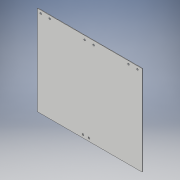
# Autodesk Inventor part: side shield
Saved by Autodesk Inventor 2017 (Build 210142000, 142)
## iProperties
Created: 2017-06-15
Part Number: side shield
Material: Generic
Document SubType Name: Modeling
Designer: slong
Density: 1 g/cm^3
Appearance: Default
Author: slong
Autodesk Inventor part; units mm, degrees
ref_plane "YZ Plane" through (0, 0, 0) normal (1, 0, 0) x (0, 1, 0)
ref_plane "XZ Plane" through (0, 0, 0) normal (0, 1, 0) x (-1, 0, 0)
ref_plane "XY Plane" through (0, 0, 0) normal (0, 0, 1) x (1, 0, 0)
sketch "Sketch1" plane through (0, 0, 0) normal (0, 0, 1) x (1, 0, 0)
  line L0 (0, -381) -> (0, 0)
  line L1 (0, 0) -> (444.5, 0)
  line L2 (444.5, 0) -> (444.5, -381)
  line L3 (444.5, -381) -> (0, -381)
  spline S0 degree 3 poles (17.3867, -12.7) (17.3867, -14.6709) (15.7889, -16.2687) (13.818, -16.2687) (11.847, -16.2687) (10.2493, -14.6709) (10.2493, -12.7) (10.2493, -10.7291) (11.847, -9.1313) (13.818, -9.1313) (15.7889, -9.1313) (17.3867, -10.7291) (17.3867, -12.7) knots 0 0 0 0 1 1 1 2 2 2 3 3 3 4 4 4 4
  line L4 (17.3867, -12.7) -> (17.3867, -14.6709) construction
  line L5 (17.3867, -14.6709) -> (15.7889, -16.2687) construction
  line L6 (15.7889, -16.2687) -> (13.818, -16.2687) construction
  line L7 (13.818, -16.2687) -> (11.847, -16.2687) construction
  line L8 (11.847, -16.2687) -> (10.2493, -14.6709) construction
  line L9 (10.2493, -14.6709) -> (10.2493, -12.7) construction
  line L10 (10.2493, -12.7) -> (10.2493, -10.7291) construction
  line L11 (10.2493, -10.7291) -> (11.847, -9.1313) construction
  line L12 (11.847, -9.1313) -> (13.818, -9.1313) construction
  line L13 (13.818, -9.1313) -> (15.7889, -9.1313) construction
  line L14 (15.7889, -9.1313) -> (17.3867, -10.7291) construction
  line L15 (17.3867, -10.7291) -> (17.3867, -12.7) construction
  spline S1 degree 3 poles (55.4867, -12.7) (55.4867, -14.6709) (53.8889, -16.2687) (51.918, -16.2687) (49.947, -16.2687) (48.3493, -14.6709) (48.3493, -12.7) (48.3493, -10.7291) (49.947, -9.1313) (51.918, -9.1313) (53.8889, -9.1313) (55.4867, -10.7291) (55.4867, -12.7) knots 0 0 0 0 1 1 1 2 2 2 3 3 3 4 4 4 4
  line L16 (55.4867, -12.7) -> (55.4867, -14.6709) construction
  line L17 (55.4867, -14.6709) -> (53.8889, -16.2687) construction
  line L18 (53.8889, -16.2687) -> (51.918, -16.2687) construction
  line L19 (51.918, -16.2687) -> (49.947, -16.2687) construction
  line L20 (49.947, -16.2687) -> (48.3493, -14.6709) construction
  line L21 (48.3493, -14.6709) -> (48.3493, -12.7) construction
  line L22 (48.3493, -12.7) -> (48.3493, -10.7291) construction
  line L23 (48.3493, -10.7291) -> (49.947, -9.1313) construction
  line L24 (49.947, -9.1313) -> (51.918, -9.1313) construction
  line L25 (51.918, -9.1313) -> (53.8889, -9.1313) construction
  line L26 (53.8889, -9.1313) -> (55.4867, -10.7291) construction
  line L27 (55.4867, -10.7291) -> (55.4867, -12.7) construction
  spline S2 degree 3 poles (390.5411, -12.7) (390.5411, -14.6709) (388.9434, -16.2687) (386.9724, -16.2687) (385.0015, -16.2687) (383.4037, -14.6709) (383.4037, -12.7) (383.4037, -10.7291) (385.0015, -9.1313) (386.9724, -9.1313) (388.9434, -9.1313) (390.5411, -10.7291) (390.5411, -12.7) knots 0 0 0 0 1 1 1 2 2 2 3 3 3 4 4 4 4
  line L28 (390.5411, -12.7) -> (390.5411, -14.6709) construction
  line L29 (390.5411, -14.6709) -> (388.9434, -16.2687) construction
  line L30 (388.9434, -16.2687) -> (386.9724, -16.2687) construction
  line L31 (386.9724, -16.2687) -> (385.0015, -16.2687) construction
  line L32 (385.0015, -16.2687) -> (383.4037, -14.6709) construction
  line L33 (383.4037, -14.6709) -> (383.4037, -12.7) construction
  line L34 (383.4037, -12.7) -> (383.4037, -10.7291) construction
  line L35 (383.4037, -10.7291) -> (385.0015, -9.1313) construction
  line L36 (385.0015, -9.1313) -> (386.9724, -9.1313) construction
  line L37 (386.9724, -9.1313) -> (388.9434, -9.1313) construction
  line L38 (388.9434, -9.1313) -> (390.5411, -10.7291) construction
  line L39 (390.5411, -10.7291) -> (390.5411, -12.7) construction
  spline S3 degree 3 poles (428.6411, -12.7) (428.6411, -14.6709) (427.0434, -16.2687) (425.0724, -16.2687) (423.1015, -16.2687) (421.5037, -14.6709) (421.5037, -12.7) (421.5037, -10.7291) (423.1015, -9.1313) (425.0724, -9.1313) (427.0434, -9.1313) (428.6411, -10.7291) (428.6411, -12.7) knots 0 0 0 0 1 1 1 2 2 2 3 3 3 4 4 4 4
  line L40 (428.6411, -12.7) -> (428.6411, -14.6709) construction
  line L41 (428.6411, -14.6709) -> (427.0434, -16.2687) construction
  line L42 (427.0434, -16.2687) -> (425.0724, -16.2687) construction
  line L43 (425.0724, -16.2687) -> (423.1015, -16.2687) construction
  line L44 (423.1015, -16.2687) -> (421.5037, -14.6709) construction
  line L45 (421.5037, -14.6709) -> (421.5037, -12.7) construction
  line L46 (421.5037, -12.7) -> (421.5037, -10.7291) construction
  line L47 (421.5037, -10.7291) -> (423.1015, -9.1313) construction
  line L48 (423.1015, -9.1313) -> (425.0724, -9.1313) construction
  line L49 (425.0724, -9.1313) -> (427.0434, -9.1313) construction
  line L50 (427.0434, -9.1313) -> (428.6411, -10.7291) construction
  line L51 (428.6411, -10.7291) -> (428.6411, -12.7) construction
  spline S4 degree 3 poles (203.9639, -16.2687) (203.9639, -18.2396) (202.3661, -19.8374) (200.3952, -19.8374) (198.4243, -19.8374) (196.8265, -18.2396) (196.8265, -16.2687) (196.8265, -14.2978) (198.4243, -12.7) (200.3952, -12.7) (202.3661, -12.7) (203.9639, -14.2978) (203.9639, -16.2687) knots 0 0 0 0 1 1 1 2 2 2 3 3 3 4 4 4 4
  line L52 (203.9639, -16.2687) -> (203.9639, -18.2396) construction
  line L53 (203.9639, -18.2396) -> (202.3661, -19.8374) construction
  line L54 (202.3661, -19.8374) -> (200.3952, -19.8374) construction
  line L55 (200.3952, -19.8374) -> (198.4243, -19.8374) construction
  line L56 (198.4243, -19.8374) -> (196.8265, -18.2396) construction
  line L57 (196.8265, -18.2396) -> (196.8265, -16.2687) construction
  line L58 (196.8265, -16.2687) -> (196.8265, -14.2978) construction
  line L59 (196.8265, -14.2978) -> (198.4243, -12.7) construction
  line L60 (198.4243, -12.7) -> (200.3952, -12.7) construction
  line L61 (200.3952, -12.7) -> (202.3661, -12.7) construction
  line L62 (202.3661, -12.7) -> (203.9639, -14.2978) construction
  line L63 (203.9639, -14.2978) -> (203.9639, -16.2687) construction
  spline S5 degree 3 poles (242.0639, -16.2687) (242.0639, -18.2396) (240.4661, -19.8374) (238.4952, -19.8374) (236.5243, -19.8374) (234.9265, -18.2396) (234.9265, -16.2687) (234.9265, -14.2978) (236.5243, -12.7) (238.4952, -12.7) (240.4661, -12.7) (242.0639, -14.2978) (242.0639, -16.2687) knots 0 0 0 0 1 1 1 2 2 2 3 3 3 4 4 4 4
  line L64 (242.0639, -16.2687) -> (242.0639, -18.2396) construction
  line L65 (242.0639, -18.2396) -> (240.4661, -19.8374) construction
  line L66 (240.4661, -19.8374) -> (238.4952, -19.8374) construction
  line L67 (238.4952, -19.8374) -> (236.5243, -19.8374) construction
  line L68 (236.5243, -19.8374) -> (234.9265, -18.2396) construction
  line L69 (234.9265, -18.2396) -> (234.9265, -16.2687) construction
  line L70 (234.9265, -16.2687) -> (234.9265, -14.2978) construction
  line L71 (234.9265, -14.2978) -> (236.5243, -12.7) construction
  line L72 (236.5243, -12.7) -> (238.4952, -12.7) construction
  line L73 (238.4952, -12.7) -> (240.4661, -12.7) construction
  line L74 (240.4661, -12.7) -> (242.0639, -14.2978) construction
  line L75 (242.0639, -14.2978) -> (242.0639, -16.2687) construction
  spline S6 degree 3 poles (197.2437, -368.3) (197.2437, -370.2709) (195.6459, -371.8687) (193.675, -371.8687) (191.7041, -371.8687) (190.1063, -370.2709) (190.1063, -368.3) (190.1063, -366.3291) (191.7041, -364.7313) (193.675, -364.7313) (195.6459, -364.7313) (197.2437, -366.3291) (197.2437, -368.3) knots 0 0 0 0 1 1 1 2 2 2 3 3 3 4 4 4 4
  line L76 (197.2437, -368.3) -> (197.2437, -370.2709) construction
  line L77 (197.2437, -370.2709) -> (195.6459, -371.8687) construction
  line L78 (195.6459, -371.8687) -> (193.675, -371.8687) construction
  line L79 (193.675, -371.8687) -> (191.7041, -371.8687) construction
  line L80 (191.7041, -371.8687) -> (190.1063, -370.2709) construction
  line L81 (190.1063, -370.2709) -> (190.1063, -368.3) construction
  line L82 (190.1063, -368.3) -> (190.1063, -366.3291) construction
  line L83 (190.1063, -366.3291) -> (191.7041, -364.7313) construction
  line L84 (191.7041, -364.7313) -> (193.675, -364.7313) construction
  line L85 (193.675, -364.7313) -> (195.6459, -364.7313) construction
  line L86 (195.6459, -364.7313) -> (197.2437, -366.3291) construction
  line L87 (197.2437, -366.3291) -> (197.2437, -368.3) construction
  spline S7 degree 3 poles (222.6437, -368.3) (222.6437, -370.2709) (221.0459, -371.8687) (219.075, -371.8687) (217.1041, -371.8687) (215.5063, -370.2709) (215.5063, -368.3) (215.5063, -366.3291) (217.1041, -364.7313) (219.075, -364.7313) (221.0459, -364.7313) (222.6437, -366.3291) (222.6437, -368.3) knots 0 0 0 0 1 1 1 2 2 2 3 3 3 4 4 4 4
  line L88 (222.6437, -368.3) -> (222.6437, -370.2709) construction
  line L89 (222.6437, -370.2709) -> (221.0459, -371.8687) construction
  line L90 (221.0459, -371.8687) -> (219.075, -371.8687) construction
  line L91 (219.075, -371.8687) -> (217.1041, -371.8687) construction
  line L92 (217.1041, -371.8687) -> (215.5063, -370.2709) construction
  line L93 (215.5063, -370.2709) -> (215.5063, -368.3) construction
  line L94 (215.5063, -368.3) -> (215.5063, -366.3291) construction
  line L95 (215.5063, -366.3291) -> (217.1041, -364.7313) construction
  line L96 (217.1041, -364.7313) -> (219.075, -364.7313) construction
  line L97 (219.075, -364.7313) -> (221.0459, -364.7313) construction
  line L98 (221.0459, -364.7313) -> (222.6437, -366.3291) construction
  line L99 (222.6437, -366.3291) -> (222.6437, -368.3) construction
  constraints: 8 end point, 1 coincident, 16 other
extrude "Extrusion1" add sketch "Sketch1" along normal blind 2.032
body "Solid1"
